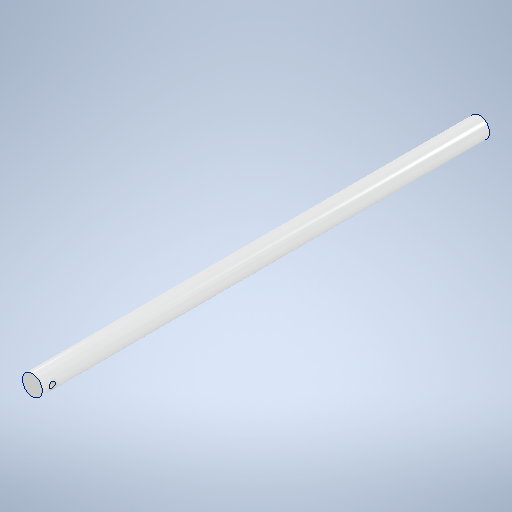
# Autodesk Inventor part: Linear Motor Bar (T-Frame)
Saved by Autodesk Inventor 2026.2 (Build 302298010, 298A)
## iProperties
Created: 2026-04-11
Part Number: Linear Motor Bar (T-Frame)
Material: Aluminum 6061
Document SubType Name: Modeling
Designer: chanh
Density: 2.7 g/cm^3
Appearance: Aluminum - Flat
Author: chanh
Autodesk Inventor part; units mm, degrees
ref_plane "YZ Plane" through (0, 0, 0) normal (1, 0, 0) x (0, 1, 0)
ref_plane "XZ Plane" through (0, 0, 0) normal (0, 1, 0) x (-1, 0, 0)
ref_plane "XY Plane" through (0, 0, 0) normal (0, 0, 1) x (1, 0, 0)
sketch "Sketch1" plane through (0, 0, 0) normal (0, 0, 1) x (1, 0, 0)
  circle A0 centre (0, 0) radius 10
  dimension "d0" = 20
  constraints: 1 centre point, 1 coincident
  measures "d0" diameter of A0
extrude "Extrusion1" add sketch "Sketch1" along normal blind 450
sketch "Sketch2" plane through (0, 0, 0) normal (1, 0, 0) x (0, 1, 0)
  line L0 (10, 450) -> (-10, 450) projected
  line L1 (10, 0) -> (-10, 0) projected
  circle A0 centre (0, 440) radius 3
  point P0 (0, 0)
  point P1 (0, 450)
  dimension "d3" = 6
  dimension "d4" = 10
  constraints: 1 centre point, 1 midpoint, 1 vertical alignment
  measures "d3" diameter of A0
  measures "d4" distance of point (0, 450) A0.centre
extrude "Extrusion2" cut sketch "Sketch2" along normal through all both and the other way through all
body "Solid1"
